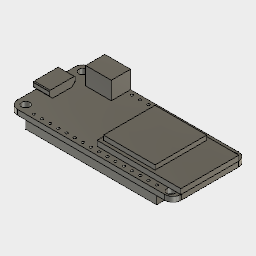
3405 ESP32 Feather HUZZAH (Autodesk Fusion 360 design; units mm, degrees)
Autodesk Fusion 360 part; units mm, degrees
sketch "Adafruit HUZZAH32 ESP32 Feather" plane through (0, 0, 0) normal (0, 0, 1) x (1, 0, 0)
  line L0 (0, 13.97) -> (0.508, 13.462)
  line L1 (0, 8.89) -> (0, 2.54)
  arc A0 (48.26, 0) -> (50.8, 2.54) centre (48.26, 2.54) ccw
  arc A1 (0, 2.54) -> (2.54, 0) centre (2.54, 2.54) ccw
  line L2 (50.8, 2.54) -> (50.8, 20.32)
  line L3 (2.54, 0) -> (48.26, 0)
  line L4 (48.26, 22.86) -> (2.54, 22.86)
  line L5 (0, 20.32) -> (0, 13.97)
  line L6 (0.508, 13.462) -> (0.508, 9.398)
  line L7 (0.508, 9.398) -> (0, 8.89)
  arc A2 (50.8, 20.32) -> (48.26, 22.86) centre (48.26, 20.32) ccw
  arc A3 (2.54, 22.86) -> (0, 20.32) centre (2.54, 20.32) ccw
  arc A4 (33.8963, 1.27) -> (34.6837, 1.27) centre (34.29, 1.27) ccw
  arc A5 (18.6563, 21.59) -> (19.4437, 21.59) centre (19.05, 21.59) ccw
  arc A6 (38.9763, 21.59) -> (39.7637, 21.59) centre (39.37, 21.59) ccw
  arc A7 (37.2237, 1.27) -> (36.4363, 1.27) centre (36.83, 1.27) ccw
  arc A8 (38.9763, 1.27) -> (39.7637, 1.27) centre (39.37, 1.27) ccw
  arc A9 (27.0637, 21.59) -> (26.2763, 21.59) centre (26.67, 21.59) ccw
  arc A10 (31.3563, 1.27) -> (32.1437, 1.27) centre (31.75, 1.27) ccw
  arc A11 (32.1437, 21.59) -> (31.3563, 21.59) centre (31.75, 21.59) ccw
  arc A12 (29.6037, 1.27) -> (28.8163, 1.27) centre (29.21, 1.27) ccw
  arc A13 (34.6837, 21.59) -> (33.8963, 21.59) centre (34.29, 21.59) ccw
  arc A14 (36.4363, 1.27) -> (37.2237, 1.27) centre (36.83, 1.27) ccw
  arc A15 (21.1963, 21.59) -> (21.9837, 21.59) centre (21.59, 21.59) ccw
  arc A16 (44.0563, 21.59) -> (44.8437, 21.59) centre (44.45, 21.59) ccw
  arc A17 (31.3563, 21.59) -> (32.1437, 21.59) centre (31.75, 21.59) ccw
  arc A18 (21.9837, 21.59) -> (21.1963, 21.59) centre (21.59, 21.59) ccw
  arc A19 (24.5237, 1.27) -> (23.7363, 1.27) centre (24.13, 1.27) ccw
  arc A20 (42.3037, 21.59) -> (41.5163, 21.59) centre (41.91, 21.59) ccw
  arc A21 (36.4363, 21.59) -> (37.2237, 21.59) centre (36.83, 21.59) ccw
  arc A22 (29.6037, 21.59) -> (28.8163, 21.59) centre (29.21, 21.59) ccw
  arc A23 (44.0563, 21.59) -> (44.8437, 21.59) centre (44.45, 21.59) ccw
  arc A24 (21.9837, 21.59) -> (21.1963, 21.59) centre (21.59, 21.59) ccw
  arc A25 (36.4363, 1.27) -> (37.2237, 1.27) centre (36.83, 1.27) ccw
  arc A26 (6.7437, 1.27) -> (5.9563, 1.27) centre (6.35, 1.27) ccw
  arc A27 (19.4437, 21.59) -> (18.6563, 21.59) centre (19.05, 21.59) ccw
  arc A28 (37.2237, 21.59) -> (36.4363, 21.59) centre (36.83, 21.59) ccw
  arc A29 (31.3563, 1.27) -> (32.1437, 1.27) centre (31.75, 1.27) ccw
  arc A30 (26.2763, 1.27) -> (27.0637, 1.27) centre (26.67, 1.27) ccw
  arc A31 (37.2237, 1.27) -> (36.4363, 1.27) centre (36.83, 1.27) ccw
  arc A32 (5.9563, 1.27) -> (6.7437, 1.27) centre (6.35, 1.27) ccw
  arc A33 (36.4363, 21.59) -> (37.2237, 21.59) centre (36.83, 21.59) ccw
  arc A34 (18.6563, 21.59) -> (19.4437, 21.59) centre (19.05, 21.59) ccw
  arc A35 (41.5163, 21.59) -> (42.3037, 21.59) centre (41.91, 21.59) ccw
  arc A36 (38.9763, 21.59) -> (39.7637, 21.59) centre (39.37, 21.59) ccw
  arc A37 (11.8237, 1.27) -> (11.0363, 1.27) centre (11.43, 1.27) ccw
  arc A38 (21.1963, 21.59) -> (21.9837, 21.59) centre (21.59, 21.59) ccw
  arc A39 (26.2763, 21.59) -> (27.0637, 21.59) centre (26.67, 21.59) ccw
  arc A40 (16.9037, 21.59) -> (16.1163, 21.59) centre (16.51, 21.59) ccw
  arc A41 (32.1437, 1.27) -> (31.3563, 1.27) centre (31.75, 1.27) ccw
  arc A42 (23.7363, 21.59) -> (24.5237, 21.59) centre (24.13, 21.59) ccw
  arc A43 (14.3637, 1.27) -> (13.5763, 1.27) centre (13.97, 1.27) ccw
  arc A44 (27.0637, 1.27) -> (26.2763, 1.27) centre (26.67, 1.27) ccw
  arc A45 (16.1163, 1.27) -> (16.9037, 1.27) centre (16.51, 1.27) ccw
  arc A46 (26.2763, 1.27) -> (27.0637, 1.27) centre (26.67, 1.27) ccw
  arc A47 (28.8163, 1.27) -> (29.6037, 1.27) centre (29.21, 1.27) ccw
  arc A48 (38.9763, 1.27) -> (39.7637, 1.27) centre (39.37, 1.27) ccw
  arc A49 (37.2237, 21.59) -> (36.4363, 21.59) centre (36.83, 21.59) ccw
  arc A50 (18.6563, 1.27) -> (19.4437, 1.27) centre (19.05, 1.27) ccw
  arc A51 (32.1437, 1.27) -> (31.3563, 1.27) centre (31.75, 1.27) ccw
  arc A52 (34.6837, 1.27) -> (33.8963, 1.27) centre (34.29, 1.27) ccw
  arc A53 (19.4437, 21.59) -> (18.6563, 21.59) centre (19.05, 21.59) ccw
  arc A54 (28.8163, 21.59) -> (29.6037, 21.59) centre (29.21, 21.59) ccw
  arc A55 (8.4963, 1.27) -> (9.2837, 1.27) centre (8.89, 1.27) ccw
  arc A56 (11.0363, 1.27) -> (11.8237, 1.27) centre (11.43, 1.27) ccw
  arc A57 (24.5237, 21.59) -> (23.7363, 21.59) centre (24.13, 21.59) ccw
  arc A58 (42.3037, 21.59) -> (41.5163, 21.59) centre (41.91, 21.59) ccw
  arc A59 (33.8963, 21.59) -> (34.6837, 21.59) centre (34.29, 21.59) ccw
  arc A60 (34.6837, 21.59) -> (33.8963, 21.59) centre (34.29, 21.59) ccw
  arc A61 (33.8963, 21.59) -> (34.6837, 21.59) centre (34.29, 21.59) ccw
  arc A62 (16.1163, 21.59) -> (16.9037, 21.59) centre (16.51, 21.59) ccw
  arc A63 (44.8437, 21.59) -> (44.0563, 21.59) centre (44.45, 21.59) ccw
  arc A64 (29.6037, 21.59) -> (28.8163, 21.59) centre (29.21, 21.59) ccw
  arc A65 (19.4437, 1.27) -> (18.6563, 1.27) centre (19.05, 1.27) ccw
  arc A66 (21.9837, 1.27) -> (21.1963, 1.27) centre (21.59, 1.27) ccw
  arc A67 (9.2837, 1.27) -> (8.4963, 1.27) centre (8.89, 1.27) ccw
  arc A68 (39.7637, 21.59) -> (38.9763, 21.59) centre (39.37, 21.59) ccw
  arc A69 (16.9037, 1.27) -> (16.1163, 1.27) centre (16.51, 1.27) ccw
  arc A70 (8.4963, 1.27) -> (9.2837, 1.27) centre (8.89, 1.27) ccw
  arc A71 (6.7437, 1.27) -> (5.9563, 1.27) centre (6.35, 1.27) ccw
  arc A72 (16.9037, 1.27) -> (16.1163, 1.27) centre (16.51, 1.27) ccw
  arc A73 (31.3563, 21.59) -> (32.1437, 21.59) centre (31.75, 21.59) ccw
  arc A74 (11.8237, 1.27) -> (11.0363, 1.27) centre (11.43, 1.27) ccw
  arc A75 (16.1163, 1.27) -> (16.9037, 1.27) centre (16.51, 1.27) ccw
  arc A76 (16.1163, 21.59) -> (16.9037, 21.59) centre (16.51, 21.59) ccw
  arc A77 (28.8163, 1.27) -> (29.6037, 1.27) centre (29.21, 1.27) ccw
  arc A78 (39.7637, 1.27) -> (38.9763, 1.27) centre (39.37, 1.27) ccw
  arc A79 (29.6037, 1.27) -> (28.8163, 1.27) centre (29.21, 1.27) ccw
  arc A80 (41.5163, 1.27) -> (42.3037, 1.27) centre (41.91, 1.27) ccw
  arc A81 (39.7637, 1.27) -> (38.9763, 1.27) centre (39.37, 1.27) ccw
  arc A82 (33.8963, 1.27) -> (34.6837, 1.27) centre (34.29, 1.27) ccw
  arc A83 (27.0637, 1.27) -> (26.2763, 1.27) centre (26.67, 1.27) ccw
  arc A84 (44.8437, 1.27) -> (44.0563, 1.27) centre (44.45, 1.27) ccw
  arc A85 (21.1963, 1.27) -> (21.9837, 1.27) centre (21.59, 1.27) ccw
  arc A86 (21.9837, 1.27) -> (21.1963, 1.27) centre (21.59, 1.27) ccw
  arc A87 (26.2763, 21.59) -> (27.0637, 21.59) centre (26.67, 21.59) ccw
  arc A88 (23.7363, 1.27) -> (24.5237, 1.27) centre (24.13, 1.27) ccw
  arc A89 (13.5763, 1.27) -> (14.3637, 1.27) centre (13.97, 1.27) ccw
  arc A90 (41.5163, 1.27) -> (42.3037, 1.27) centre (41.91, 1.27) ccw
  arc A91 (24.5237, 1.27) -> (23.7363, 1.27) centre (24.13, 1.27) ccw
  arc A92 (19.4437, 1.27) -> (18.6563, 1.27) centre (19.05, 1.27) ccw
  arc A93 (14.3637, 1.27) -> (13.5763, 1.27) centre (13.97, 1.27) ccw
  arc A94 (42.3037, 1.27) -> (41.5163, 1.27) centre (41.91, 1.27) ccw
  arc A95 (18.6563, 1.27) -> (19.4437, 1.27) centre (19.05, 1.27) ccw
  arc A96 (34.6837, 1.27) -> (33.8963, 1.27) centre (34.29, 1.27) ccw
  arc A97 (16.9037, 21.59) -> (16.1163, 21.59) centre (16.51, 21.59) ccw
  arc A98 (39.7637, 21.59) -> (38.9763, 21.59) centre (39.37, 21.59) ccw
  arc A99 (5.9563, 1.27) -> (6.7437, 1.27) centre (6.35, 1.27) ccw
  arc A100 (24.5237, 21.59) -> (23.7363, 21.59) centre (24.13, 21.59) ccw
  arc A101 (9.2837, 1.27) -> (8.4963, 1.27) centre (8.89, 1.27) ccw
  arc A102 (44.8437, 21.59) -> (44.0563, 21.59) centre (44.45, 21.59) ccw
  arc A103 (28.8163, 21.59) -> (29.6037, 21.59) centre (29.21, 21.59) ccw
  arc A104 (41.5163, 21.59) -> (42.3037, 21.59) centre (41.91, 21.59) ccw
  arc A105 (44.8437, 1.27) -> (44.0563, 1.27) centre (44.45, 1.27) ccw
  arc A106 (11.0363, 1.27) -> (11.8237, 1.27) centre (11.43, 1.27) ccw
  arc A107 (13.5763, 1.27) -> (14.3637, 1.27) centre (13.97, 1.27) ccw
  arc A108 (44.0563, 1.27) -> (44.8437, 1.27) centre (44.45, 1.27) ccw
  arc A109 (32.1437, 21.59) -> (31.3563, 21.59) centre (31.75, 21.59) ccw
  arc A110 (44.0563, 1.27) -> (44.8437, 1.27) centre (44.45, 1.27) ccw
  arc A111 (21.1963, 1.27) -> (21.9837, 1.27) centre (21.59, 1.27) ccw
  arc A112 (42.3037, 1.27) -> (41.5163, 1.27) centre (41.91, 1.27) ccw
  arc A113 (23.7363, 21.59) -> (24.5237, 21.59) centre (24.13, 21.59) ccw
  arc A114 (27.0637, 21.59) -> (26.2763, 21.59) centre (26.67, 21.59) ccw
  arc A115 (23.7363, 1.27) -> (24.5237, 1.27) centre (24.13, 1.27) ccw
  circle A116 centre (2.54, 2.54) radius 1.27
  circle A117 centre (2.54, 20.32) radius 1.27
  circle A118 centre (48.26, 20.955) radius 1.27
  circle A119 centre (48.26, 1.8415) radius 1.27
  dimension "d1" = 2.54
  dimension "d2" = 2.54
  dimension "d3" = 2.54
  dimension "d4" = 2.54
  measures "d1" diameter of A116
  measures "d2" diameter of A117
  measures "d3" diameter of A118
  measures "d4" diameter of A119
extrude "Extrude1" add sketch "Adafruit HUZZAH32 ESP32 Feather" along normal blind 1.6 makes body 1
sketch "microUSB" plane through (0, 0, 1.6) normal (0, 0, 1) x (-1, 0, 0)
  circle A0 centre (-16.51, -21.59) radius 0.3937
  circle A1 centre (-39.37, -21.59) radius 0.3937
  circle A2 centre (-21.59, -1.27) radius 0.3937
  circle A3 centre (-39.37, -1.27) radius 0.3937
  circle A4 centre (-13.97, -1.27) radius 0.3937
  circle A5 centre (-6.35, -1.27) radius 0.3937
  circle A6 centre (-11.43, -1.27) radius 0.3937
  circle A7 centre (-44.45, -1.27) radius 0.3937
  circle A8 centre (-31.75, -21.59) radius 0.3937
  circle A9 centre (-2.54, -20.32) radius 1.27
  circle A10 centre (-48.26, -20.955) radius 1.27
  circle A11 centre (-24.13, -21.59) radius 0.3937
  circle A12 centre (-41.91, -21.59) radius 0.3937
  circle A13 centre (-24.13, -1.27) radius 0.3937
  circle A14 centre (-26.67, -1.27) radius 0.3937
  circle A15 centre (-26.67, -21.59) radius 0.3937
  circle A16 centre (-2.54, -2.54) radius 1.27
  circle A17 centre (-19.05, -1.27) radius 0.3937
  circle A18 centre (-16.51, -1.27) radius 0.3937
  circle A19 centre (-36.83, -21.59) radius 0.3937
  circle A20 centre (-48.26, -1.8415) radius 1.27
  circle A21 centre (-34.29, -21.59) radius 0.3937
  circle A22 centre (-44.45, -21.59) radius 0.3937
  circle A23 centre (-34.29, -1.27) radius 0.3937
  circle A24 centre (-41.91, -1.27) radius 0.3937
  circle A25 centre (-29.21, -1.27) radius 0.3937
  circle A26 centre (-19.05, -21.59) radius 0.3937
  circle A27 centre (-29.21, -21.59) radius 0.3937
  circle A28 centre (-8.89, -1.27) radius 0.3937
  circle A29 centre (-36.83, -1.27) radius 0.3937
  circle A30 centre (-21.59, -21.59) radius 0.3937
  circle A31 centre (-31.75, -1.27) radius 0.3937
  arc A32 (-2.54, -22.86) -> (0, -20.32) centre (-2.54, -20.32) ccw
  line L0 (0, -20.32) -> (0, -13.97)
  line L1 (0, -13.97) -> (-0.508, -13.462)
  line L2 (-0.508, -13.462) -> (-0.508, -9.398)
  line L3 (-0.508, -9.398) -> (0, -8.89)
  line L4 (0, -8.89) -> (0, -2.54)
  arc A33 (0, -2.54) -> (-2.54, 0) centre (-2.54, -2.54) ccw
  line L5 (-2.54, 0) -> (-48.26, 0)
  arc A34 (-48.26, 0) -> (-50.8, -2.54) centre (-48.26, -2.54) ccw
  line L6 (-50.8, -2.54) -> (-50.8, -20.32)
  arc A35 (-50.8, -20.32) -> (-48.26, -22.86) centre (-48.26, -20.32) ccw
  line L7 (-48.26, -22.86) -> (-2.54, -22.86)
  line L8 (0, -15.43) -> (-5, -15.43)
  line L9 (-5, -15.43) -> (-5, -7.43)
  line L10 (-5, -7.43) -> (0, -7.43)
  line L11 (0, -7.43) -> (0, -15.43)
  line L12 (0, -11.43) -> (-0.508, -11.43) construction
  dimension "d7" = 5
  dimension "d8" = 8
  measures "d7" distance of L8.start L8.end
  measures "d8" distance of L8.start L10.end
extrude "Extrude2" add sketch "microUSB" along normal blind 2.5 separate body contours L0 L1 L2 L3 L4 L8 L9 L10 L11 | L1 L2 L3 L11 makes body 2
chamfer "Chamfer1" distance 1 angle 45 2 edges at (2.5, 15.43, 1.6) (2.5, 7.43, 1.6) on bodies 2
fillet "Fillet1" radius 0.25 6 edges at (2.5, 15.43, 4.1) (2.5, 15.43, 2.6) (2.5, 14.43, 1.6) (2.5, 8.43, 1.6) (2.5, 7.43, 2.6) (2.5, 7.43, 4.1) on bodies 2
shell "Shell1" thickness 0.4 removed faces 1 at (0, 10.4645, 3.2667) on bodies 2
sketch "JST" plane through (0, 0, 1.6) normal (0, 0, 1) x (-1, 0, 0)
  circle A0 centre (-16.51, -21.59) radius 0.3937
  circle A1 centre (-39.37, -21.59) radius 0.3937
  circle A2 centre (-21.59, -1.27) radius 0.3937
  circle A3 centre (-39.37, -1.27) radius 0.3937
  circle A4 centre (-13.97, -1.27) radius 0.3937
  circle A5 centre (-6.35, -1.27) radius 0.3937
  circle A6 centre (-11.43, -1.27) radius 0.3937
  circle A7 centre (-44.45, -1.27) radius 0.3937
  circle A8 centre (-31.75, -21.59) radius 0.3937
  circle A9 centre (-2.54, -20.32) radius 1.27
  circle A10 centre (-48.26, -20.955) radius 1.27
  circle A11 centre (-24.13, -21.59) radius 0.3937
  circle A12 centre (-41.91, -21.59) radius 0.3937
  circle A13 centre (-24.13, -1.27) radius 0.3937
  circle A14 centre (-26.67, -1.27) radius 0.3937
  circle A15 centre (-26.67, -21.59) radius 0.3937
  circle A16 centre (-2.54, -2.54) radius 1.27
  circle A17 centre (-19.05, -1.27) radius 0.3937
  circle A18 centre (-16.51, -1.27) radius 0.3937
  circle A19 centre (-36.83, -21.59) radius 0.3937
  circle A20 centre (-48.26, -1.8415) radius 1.27
  circle A21 centre (-34.29, -21.59) radius 0.3937
  circle A22 centre (-44.45, -21.59) radius 0.3937
  circle A23 centre (-34.29, -1.27) radius 0.3937
  circle A24 centre (-41.91, -1.27) radius 0.3937
  circle A25 centre (-29.21, -1.27) radius 0.3937
  circle A26 centre (-19.05, -21.59) radius 0.3937
  circle A27 centre (-29.21, -21.59) radius 0.3937
  circle A28 centre (-8.89, -1.27) radius 0.3937
  circle A29 centre (-36.83, -1.27) radius 0.3937
  circle A30 centre (-21.59, -21.59) radius 0.3937
  circle A31 centre (-31.75, -1.27) radius 0.3937
  arc A32 (-2.54, -22.86) -> (0, -20.32) centre (-2.54, -20.32) ccw
  line L0 (0, -20.32) -> (0, -13.97)
  line L1 (0, -13.97) -> (-0.508, -13.462)
  line L2 (-0.508, -13.462) -> (-0.508, -9.398)
  line L3 (-0.508, -9.398) -> (0, -8.89)
  line L4 (0, -8.89) -> (0, -2.54)
  arc A33 (0, -2.54) -> (-2.54, 0) centre (-2.54, -2.54) ccw
  line L5 (-2.54, 0) -> (-48.26, 0)
  arc A34 (-48.26, 0) -> (-50.8, -2.54) centre (-48.26, -2.54) ccw
  line L6 (-50.8, -2.54) -> (-50.8, -20.32)
  arc A35 (-50.8, -20.32) -> (-48.26, -22.86) centre (-48.26, -20.32) ccw
  line L7 (-48.26, -22.86) -> (-2.54, -22.86)
  line L8 (-6.795, -22.86) -> (-14.795, -22.86)
  line L9 (-14.795, -22.86) -> (-14.795, -16.86)
  line L10 (-14.795, -16.86) -> (-6.795, -16.86)
  line L11 (-6.795, -16.86) -> (-6.795, -22.86)
  line L12 (-10.795, -22.86) -> (-10.795, -16.86) construction
  dimension "d14" = 8
  dimension "d15" = 6
  dimension "d16" = 10.795
  measures "d14" distance of L8.start L8.end
  measures "d15" distance of L8.start L10.end
  measures "d16" distance of L0 L12
extrude "Extrude3" add sketch "JST" along normal blind 5.5 separate body contours L7 L8 L9 L10 L11 makes body 3
sketch "ESP32 PCB" plane through (0, 0, 1.6) normal (0, 0, 1) x (-1, 0, 0)
  circle A0 centre (-16.51, -21.59) radius 0.3937
  circle A1 centre (-39.37, -21.59) radius 0.3937
  circle A2 centre (-21.59, -1.27) radius 0.3937
  circle A3 centre (-39.37, -1.27) radius 0.3937
  circle A4 centre (-13.97, -1.27) radius 0.3937
  circle A5 centre (-6.35, -1.27) radius 0.3937
  circle A6 centre (-11.43, -1.27) radius 0.3937
  circle A7 centre (-44.45, -1.27) radius 0.3937
  circle A8 centre (-31.75, -21.59) radius 0.3937
  circle A9 centre (-2.54, -20.32) radius 1.27
  circle A10 centre (-48.26, -20.955) radius 1.27 construction
  circle A11 centre (-24.13, -21.59) radius 0.3937
  circle A12 centre (-41.91, -21.59) radius 0.3937
  circle A13 centre (-24.13, -1.27) radius 0.3937
  circle A14 centre (-26.67, -1.27) radius 0.3937
  circle A15 centre (-26.67, -21.59) radius 0.3937
  circle A16 centre (-2.54, -2.54) radius 1.27
  circle A17 centre (-19.05, -1.27) radius 0.3937
  circle A18 centre (-16.51, -1.27) radius 0.3937
  circle A19 centre (-36.83, -21.59) radius 0.3937
  circle A20 centre (-48.26, -1.8415) radius 1.27 construction
  circle A21 centre (-34.29, -21.59) radius 0.3937
  circle A22 centre (-44.45, -21.59) radius 0.3937
  circle A23 centre (-34.29, -1.27) radius 0.3937
  circle A24 centre (-41.91, -1.27) radius 0.3937
  circle A25 centre (-29.21, -1.27) radius 0.3937
  circle A26 centre (-19.05, -21.59) radius 0.3937
  circle A27 centre (-29.21, -21.59) radius 0.3937
  circle A28 centre (-8.89, -1.27) radius 0.3937
  circle A29 centre (-36.83, -1.27) radius 0.3937
  circle A30 centre (-21.59, -21.59) radius 0.3937
  circle A31 centre (-31.75, -1.27) radius 0.3937
  arc A32 (-2.54, -22.86) -> (0, -20.32) centre (-2.54, -20.32) ccw
  line L0 (0, -20.32) -> (0, -13.97)
  line L1 (0, -13.97) -> (-0.508, -13.462)
  line L2 (-0.508, -13.462) -> (-0.508, -9.398)
  line L3 (-0.508, -9.398) -> (0, -8.89)
  line L4 (0, -8.89) -> (0, -2.54)
  arc A33 (0, -2.54) -> (-2.54, 0) centre (-2.54, -2.54) ccw
  line L5 (-2.54, 0) -> (-48.26, 0)
  arc A34 (-48.26, 0) -> (-50.8, -2.54) centre (-48.26, -2.54) ccw construction
  line L6 (-50.8, -2.54) -> (-50.8, -20.32)
  arc A35 (-50.8, -20.32) -> (-48.26, -22.86) centre (-48.26, -20.32) ccw construction
  line L7 (-48.26, -22.86) -> (-2.54, -22.86)
  line L8 (-50.8, -2.43) -> (-24.8, -2.43)
  line L9 (-24.8, -2.43) -> (-24.8, -20.43)
  line L10 (-24.8, -20.43) -> (-50.8, -20.43)
  line L11 (-50.8, -20.43) -> (-50.8, -2.43)
  line L12 (-50.8, -2.43) -> (-24.8, -20.43) construction
  line L13 (-24.8, -2.43) -> (-50.8, -20.43) construction
  point P0 (-37.8, -11.43)
  dimension "d19" = 26
  dimension "d20" = 18
  dimension "d21" = 11.43
  measures "d19" distance of L9.end L10.end
  measures "d20" distance of L8.end L9.end
  measures "d21" distance of L5 P0
extrude "Extrude4" add sketch "ESP32 PCB" along normal blind 1.6 separate body contours L6 L8 L9 L10 L11 makes body 4
sketch "ESP32 IC" plane through (0, 0, 3.2) normal (0, 0, 1) x (-1, 0, 0)
  line L0 (-50.8, -20.43) -> (-24.8, -20.43)
  line L1 (-24.8, -20.43) -> (-24.8, -2.43)
  line L2 (-24.8, -2.43) -> (-50.8, -2.43)
  line L3 (-50.8, -2.43) -> (-50.8, -20.43)
  line L4 (-25.8, -19.43) -> (-41.8, -19.43)
  line L5 (-41.8, -19.43) -> (-41.8, -3.43)
  line L6 (-41.8, -3.43) -> (-25.8, -3.43)
  line L7 (-25.8, -3.43) -> (-25.8, -19.43)
  dimension "d25" = 1
  dimension "d26" = 1
  dimension "d27" = 1
  dimension "d28" = 16
  measures "d25" distance of L2 L6
  measures "d26" distance of L1 L7
  measures "d27" distance of L0 L4
  measures "d28" distance of L5 L7
extrude "Extrude5" add sketch "ESP32 IC" along normal blind 1.4 contours L4 L5 L6 L7 bodies 4
sketch "header pins" plane through (0, 0, 0) normal (0, 0, -1) x (1, 0, 0)
  circle A0 centre (16.51, -21.59) radius 0.3937
  circle A1 centre (39.37, -21.59) radius 0.3937
  circle A2 centre (21.59, -1.27) radius 0.3937
  circle A3 centre (39.37, -1.27) radius 0.3937
  circle A4 centre (13.97, -1.27) radius 0.3937
  circle A5 centre (6.35, -1.27) radius 0.3937
  circle A6 centre (11.43, -1.27) radius 0.3937
  circle A7 centre (44.45, -1.27) radius 0.3937
  circle A8 centre (31.75, -21.59) radius 0.3937
  circle A9 centre (2.54, -20.32) radius 1.27
  circle A10 centre (48.26, -20.955) radius 1.27
  circle A11 centre (24.13, -21.59) radius 0.3937
  circle A12 centre (41.91, -21.59) radius 0.3937
  circle A13 centre (24.13, -1.27) radius 0.3937
  circle A14 centre (26.67, -1.27) radius 0.3937
  circle A15 centre (26.67, -21.59) radius 0.3937
  circle A16 centre (2.54, -2.54) radius 1.27
  circle A17 centre (19.05, -1.27) radius 0.3937
  circle A18 centre (16.51, -1.27) radius 0.3937
  circle A19 centre (36.83, -21.59) radius 0.3937
  circle A20 centre (48.26, -1.8415) radius 1.27
  circle A21 centre (34.29, -21.59) radius 0.3937
  circle A22 centre (44.45, -21.59) radius 0.3937
  circle A23 centre (34.29, -1.27) radius 0.3937
  circle A24 centre (41.91, -1.27) radius 0.3937
  circle A25 centre (29.21, -1.27) radius 0.3937
  circle A26 centre (19.05, -21.59) radius 0.3937
  circle A27 centre (29.21, -21.59) radius 0.3937
  circle A28 centre (8.89, -1.27) radius 0.3937
  circle A29 centre (36.83, -1.27) radius 0.3937
  circle A30 centre (21.59, -21.59) radius 0.3937
  circle A31 centre (31.75, -1.27) radius 0.3937
  arc A32 (0, -20.32) -> (2.54, -22.86) centre (2.54, -20.32) ccw
  line L0 (2.54, -22.86) -> (48.26, -22.86)
  arc A33 (48.26, -22.86) -> (50.8, -20.32) centre (48.26, -20.32) ccw
  line L1 (50.8, -20.32) -> (50.8, -2.54)
  arc A34 (50.8, -2.54) -> (48.26, 0) centre (48.26, -2.54) ccw
  line L2 (48.26, 0) -> (2.54, 0)
  arc A35 (2.54, 0) -> (0, -2.54) centre (2.54, -2.54) ccw
  line L3 (0, -2.54) -> (0, -8.89)
  line L4 (0, -8.89) -> (0.508, -9.398)
  line L5 (0.508, -9.398) -> (0.508, -13.462)
  line L6 (0.508, -13.462) -> (0, -13.97)
  line L7 (0, -13.97) -> (0, -20.32)
  line L8 (45.72, 0) -> (5.08, 0)
  line L9 (5.08, 0) -> (5.08, -2.54)
  line L10 (5.08, -2.54) -> (45.72, -2.54)
  line L11 (45.72, -2.54) -> (45.72, 0)
  line L12 (45.72, -20.32) -> (15.24, -20.32)
  line L13 (15.24, -20.32) -> (15.24, -22.86)
  line L14 (15.24, -22.86) -> (45.72, -22.86)
  line L15 (45.72, -22.86) -> (45.72, -20.32)
  dimension "d31" = 1.27
  dimension "d32" = 1.27
  dimension "d33" = 1.27
  dimension "d34" = 1.27
  dimension "d35" = 1.27
  dimension "d36" = 1.27
  measures "d31" distance of A5.centre L10
  measures "d32" distance of A5.centre L9
  measures "d33" distance of A7.centre L11
  measures "d34" distance of A0.centre L13
  measures "d35" distance of A0.centre L12
  measures "d36" distance of A22.centre L15
extrude "Extrude6" add sketch "header pins" along normal blind 2.5 separate body contours L0 L12 L13 L14 L15 | L2 L8 L9 L10 L11 makes body 5 at (32.1733, 0, -1.6667) makes body 6 at (35.56, 20.32, -0.8333)
named bodies: "PCB", "microUSB", "JST", "ESP32"
